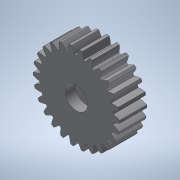
# Autodesk Inventor part: small-gear
Saved by Autodesk Inventor 2020 (Build 240168000, 168)
## iProperties
Created: 2020-05-22
Part Number: small-gear
Material: Ogólny
Document SubType Name: Modeling
Designer: blep
Density: 1 g/cm^3
Appearance: Domyślna
Author: blep
Autodesk Inventor part; units mm, degrees
ref_plane "YZ Plane" through (0, 0, 0) normal (1, 0, 0) x (0, 1, 0)
ref_plane "XZ Plane" through (0, 0, 0) normal (0, 1, 0) x (-1, 0, 0)
ref_plane "XY Plane" through (0, 0, 0) normal (0, 0, 1) x (1, 0, 0)
sketch "Szkic1" plane through (0, 0, 0) normal (0, 0, 1) x (1, 0, 0)
  arc A0 (-1.732, -4.0613) -> (-1.6613, -4.132) centre (0, -2.4) ccw projected
  arc A1 (0.05, -0.4006) -> (-0.05, -0.4006) centre (0, -2.4) ccw projected
  arc A2 (-0.05, -0.4006) -> (-0.5703, -0.483) centre (0, -2.4) ccw projected
  arc A3 (-0.5703, -0.483) -> (-0.6654, -0.5139) centre (0, -2.4) ccw projected
  arc A4 (-0.6654, -0.5139) -> (-1.1348, -0.7531) centre (0, -2.4) ccw projected
  arc A5 (-1.1348, -0.7531) -> (-1.2157, -0.8119) centre (0, -2.4) ccw projected
  arc A6 (-1.2157, -0.8119) -> (-1.5881, -1.1843) centre (0, -2.4) ccw projected
  arc A7 (-1.5881, -1.1843) -> (-1.6469, -1.2652) centre (0, -2.4) ccw projected
  arc A8 (-1.6469, -1.2652) -> (-1.8861, -1.7346) centre (0, -2.4) ccw projected
  arc A9 (-1.8861, -1.7346) -> (-1.917, -1.8297) centre (0, -2.4) ccw projected
  arc A10 (-1.917, -1.8297) -> (-1.9994, -2.35) centre (0, -2.4) ccw projected
  arc A11 (-1.9994, -2.35) -> (-1.9994, -2.45) centre (0, -2.4) ccw projected
  arc A12 (-1.9994, -2.45) -> (-1.917, -2.9703) centre (0, -2.4) ccw projected
  arc A13 (-1.917, -2.9703) -> (-1.8861, -3.0654) centre (0, -2.4) ccw projected
  arc A14 (-1.8861, -3.0654) -> (-1.6469, -3.5348) centre (0, -2.4) ccw projected
  arc A15 (-1.6469, -3.5348) -> (-1.5881, -3.6157) centre (0, -2.4) ccw projected
  arc A16 (-1.5881, -3.6157) -> (-1.2157, -3.9881) centre (0, -2.4) ccw projected
  arc A17 (-1.2157, -3.9881) -> (-1.1348, -4.0469) centre (0, -2.4) ccw projected
  arc A18 (-1.1348, -4.0469) -> (-0.6654, -4.2861) centre (0, -2.4) ccw projected
  arc A19 (-0.6654, -4.2861) -> (-0.5703, -4.317) centre (0, -2.4) ccw projected
  arc A20 (-0.5703, -4.317) -> (-0.05, -4.3994) centre (0, -2.4) ccw projected
  arc A21 (-0.05, -4.3994) -> (0.05, -4.3994) centre (0, -2.4) ccw projected
  arc A22 (0.05, -4.3994) -> (0.5703, -4.317) centre (0, -2.4) ccw projected
  arc A23 (0.5703, -4.317) -> (0.6654, -4.2861) centre (0, -2.4) ccw projected
  arc A24 (0.6654, -4.2861) -> (1.1348, -4.0469) centre (0, -2.4) ccw projected
  arc A25 (1.1348, -4.0469) -> (1.2157, -3.9881) centre (0, -2.4) ccw projected
  arc A26 (1.2157, -3.9881) -> (1.5881, -3.6157) centre (0, -2.4) ccw projected
  arc A27 (1.5881, -3.6157) -> (1.6469, -3.5348) centre (0, -2.4) ccw projected
  arc A28 (1.6469, -3.5348) -> (1.8861, -3.0654) centre (0, -2.4) ccw projected
  arc A29 (1.8861, -3.0654) -> (1.917, -2.9703) centre (0, -2.4) ccw projected
  arc A30 (1.917, -2.9703) -> (1.9994, -2.45) centre (0, -2.4) ccw projected
  arc A31 (1.9994, -2.45) -> (1.9994, -2.35) centre (0, -2.4) ccw projected
  arc A32 (1.9994, -2.35) -> (1.917, -1.8297) centre (0, -2.4) ccw projected
  arc A33 (1.917, -1.8297) -> (1.8861, -1.7346) centre (0, -2.4) ccw projected
  arc A34 (1.8861, -1.7346) -> (1.6469, -1.2652) centre (0, -2.4) ccw projected
  arc A35 (1.6469, -1.2652) -> (1.5881, -1.1843) centre (0, -2.4) ccw projected
  arc A36 (1.5881, -1.1843) -> (1.2157, -0.8119) centre (0, -2.4) ccw projected
  arc A37 (1.2157, -0.8119) -> (1.1348, -0.7531) centre (0, -2.4) ccw projected
  arc A38 (1.1348, -0.7531) -> (0.6654, -0.5139) centre (0, -2.4) ccw projected
  arc A39 (0.6654, -0.5139) -> (0.5703, -0.483) centre (0, -2.4) ccw projected
  arc A40 (0.5703, -0.483) -> (0.05, -0.4006) centre (0, -2.4) ccw projected
  circle A41 centre (0, -2.4) radius 1.5065 projected
  circle A42 centre (0, -2.4) radius 2.4
  circle A43 centre (0, -2.4) radius 15
  circle A44 centre (0, -2.4) radius 1.0065 projected
  circle A45 centre (0, -2.4) radius 1.2565
  circle A46 centre (0, -2.4) radius 2.9
  point P0 (0, 0)
  point P1 (-1.6613, -4.132)
  point P2 (-1.732, -4.0613)
  dimension "d0" = 30
  dimension "d3" = 0.25
  dimension "d12" = 0.5
  constraints: 4 centre point, 2 coincident, 1 concentric
  measures "d0" diameter of A43
  measures "d3" radial gap between concentric circles of A44 A45
  measures "d12" radial gap between concentric circles of A42 A46
extrude "Wyciągnięcie proste1" add sketch "Szkic1" against normal blind 3 contours A43
extrude "Wyciągnięcie proste2" add sketch "Szkic1" along normal blind 1.5 contours A42 A0 | A40 A39 A38 A37 A36 A35 A34 A33 A32 A31 A30 A29 A28 A27 A26 A25 A24 A23 A22 A21 A20 A19 A18 A17 A16 A15 A14 A13 A12 A11 A10 A9 A8 A7 A6 A5 A4 A3 A2 A1 | A41 | A43 | A45 | A46
sketch "Szkic2" plane through (0, -2.4, 1.5) normal (0, 0, 1) x (1, 0, 0)
  circle A0 centre (0, 0) radius 1.0065 projected
  circle A1 centre (0, 0) radius 3
  circle A2 centre (0, 0) radius 15 projected
  point P0 (0, 2.4)
  dimension "d6" = 6
  constraints: 1 centre point, 1 coincident
  measures "d6" diameter of A1
extrude "Wyciągnięcie proste3" add sketch "Szkic2" along normal blind 2.7 contours A2
sketch "Szkic4" plane through (0, -2.4, -3) normal (0, 0, -1) x (-1, 0, 0)
  arc A0 (4.4308, -8.6273) -> (5.208, -8.1816) centre (0, 0) ccw projected
  arc A1 (1.0151, -9.6453) -> (1.9007, -9.5105) centre (0, 0) ccw projected
  arc A2 (-2.5377, -9.3607) -> (-1.6632, -9.5549) centre (0, 0) ccw projected
  arc A3 (-5.7478, -7.8118) -> (-5.0025, -8.3088) centre (0, 0) ccw projected
  arc A4 (-8.1816, -5.208) -> (-7.6662, -5.9407) centre (0, 0) ccw projected
  arc A5 (-9.5105, -1.9007) -> (-9.2945, -2.7701) centre (0, 0) ccw projected
  arc A6 (-9.5549, 1.6632) -> (-9.6676, 0.7745) centre (0, 0) ccw projected
  arc A7 (-8.3088, 5.0025) -> (-8.735, 4.2145) centre (0, 0) ccw projected
  arc A8 (-5.9407, 7.6662) -> (-6.6227, 7.0854) centre (0, 0) ccw projected
  arc A9 (7.8118, -5.7478) -> (6.4204, -3.8655) centre (1.2511, -9.1422) ccw projected
  arc A10 (6.4204, -3.8655) -> (6.7497, -3.2567) centre (0, 0) ccw projected
  arc A11 (6.7497, -3.2567) -> (9.0866, -3.3906) centre (8.3355, 3.958) ccw projected
  arc A12 (9.0866, -3.3906) -> (9.3607, -2.5377) centre (0, 0) ccw projected
  arc A13 (9.3607, -2.5377) -> (7.3833, -1.2852) centre (4.4691, -8.0729) ccw projected
  arc A14 (7.3833, -1.2852) -> (7.4703, -0.5985) centre (0, 0) ccw projected
  arc A15 (7.4703, -0.5985) -> (9.6978, 0.1208) centre (6.3428, 6.7018) ccw projected
  arc A16 (9.6978, 0.1208) -> (9.6453, 1.0151) centre (0, 0) ccw projected
  arc A17 (9.6453, 1.0151) -> (7.3489, 1.4687) centre (7.0836, -5.9134) ccw projected
  arc A18 (7.3489, 1.4687) -> (7.1821, 2.1405) centre (0, 0) ccw projected
  arc A19 (7.1821, 2.1405) -> (8.9993, 3.6159) centre (3.4935, 8.5406) ccw projected
  arc A20 (8.9993, 3.6159) -> (8.6273, 4.4308) centre (0, 0) ccw projected
  arc A21 (8.6273, 4.4308) -> (6.3221, 4.0243) centre (8.7414, -2.9551) ccw projected
  arc A22 (6.3221, 4.0243) -> (5.9238, 4.5905) centre (0, 0) ccw projected
  arc A23 (5.9238, 4.5905) -> (7.0854, 6.6227) centre (0.1724, 9.2258) ccw projected
  arc A24 (7.0854, 6.6227) -> (6.4441, 7.2482) centre (0, 0) ccw projected
  arc A25 (6.4441, 7.2482) -> (4.4415, 6.0364) centre (9.2187, 0.4022) ccw projected
  arc A26 (4.4415, 6.0364) -> (3.8655, 6.4204) centre (0, 0) ccw projected
  arc A27 (3.8655, 6.4204) -> (4.2145, 8.735) centre (-3.172, 8.6651) ccw projected
  arc A28 (4.2145, 8.735) -> (3.3906, 9.0866) centre (0, 0) ccw projected
  arc A29 (3.3906, 9.0866) -> (1.9609, 7.2332) centre (8.4509, 3.7052) ccw projected
  arc A30 (1.9609, 7.2332) -> (1.2852, 7.3833) centre (0, 0) ccw projected
  arc A31 (1.2852, 7.3833) -> (0.7745, 9.6676) centre (-6.088, 6.9341) ccw projected
  arc A32 (0.7745, 9.6676) -> (-0.1208, 9.6978) centre (0, 0) ccw projected
  arc A33 (-0.1208, 9.6978) -> (-0.7844, 7.4531) centre (6.5417, 6.5078) ccw projected
  arc A34 (-0.7844, 7.4531) -> (-1.4687, 7.3489) centre (0, 0) ccw projected
  arc A35 (-1.4687, 7.3489) -> (-2.7701, 9.2945) centre (-8.1818, 4.2666) ccw projected
  arc A36 (-2.7701, 9.2945) -> (-3.6159, 8.9993) centre (0, 0) ccw projected
  arc A37 (-3.6159, 8.9993) -> (-3.4238, 6.6665) centre (3.7491, 8.4315) ccw projected
  arc A38 (-3.4238, 6.6665) -> (-4.0243, 6.3221) centre (0, 0) ccw projected
  arc A39 (-4.0243, 6.3221) -> (-5.9407, 7.6662) centre (-9.1706, 1.0229) ccw projected
  arc A40 (-6.6227, 7.0854) -> (-5.6008, 4.9795) centre (0.4501, 9.2165) ccw projected
  arc A41 (-5.6008, 4.9795) -> (-6.0364, 4.4415) centre (0, 0) ccw projected
  arc A42 (-6.0364, 4.4415) -> (-8.3088, 5.0025) centre (-8.9208, -2.359) ccw projected
  arc A43 (-8.735, 4.2145) -> (-7.0214, 2.62) centre (-2.9097, 8.7567) ccw projected
  arc A44 (-7.0214, 2.62) -> (-7.2332, 1.9609) centre (0, 0) ccw projected
  arc A45 (-7.2332, 1.9609) -> (-9.5549, 1.6632) centre (-7.4663, -5.4222) ccw projected
  arc A46 (-9.6676, 0.7745) -> (-7.4937, -0.0934) centre (-5.8765, 7.1143) ccw projected
  arc A47 (-7.4937, -0.0934) -> (-7.4531, -0.7844) centre (0, 0) ccw projected
  arc A48 (-7.4531, -0.7844) -> (-9.5105, -1.9007) centre (-5.0034, -7.7532) ccw projected
  arc A49 (-9.2945, -2.7701) -> (-6.9539, -2.7941) centre (-8.0496, 4.5111) ccw projected
  arc A50 (-6.9539, -2.7941) -> (-6.6665, -3.4238) centre (0, 0) ccw projected
  arc A51 (-6.6665, -3.4238) -> (-8.1816, -5.208) centre (-1.8647, -9.0371) ccw projected
  arc A52 (-7.6662, -5.9407) -> (-5.475, -5.1175) centre (-9.1356, 1.2986) ccw projected
  arc A53 (-5.475, -5.1175) -> (-4.9795, -5.6008) centre (0, 0) ccw projected
  arc A54 (-4.9795, -5.6008) -> (-5.7478, -7.8118) centre (1.5258, -9.1004) ccw projected
  arc A55 (-5.0025, -8.3088) -> (-3.2567, -6.7497) centre (-8.9878, -2.0893) ccw projected
  arc A56 (-3.2567, -6.7497) -> (-2.62, -7.0214) centre (0, 0) ccw projected
  arc A57 (-2.62, -7.0214) -> (-2.5377, -9.3607) centre (4.7102, -7.9347) ccw projected
  arc A58 (-1.6632, -9.5549) -> (-0.5985, -7.4703) centre (-7.6261, -5.195) ccw projected
  arc A59 (-0.5985, -7.4703) -> (0.0934, -7.4937) centre (0, 0) ccw projected
  arc A60 (0.0934, -7.4937) -> (1.0151, -9.6453) centre (7.2585, -5.6974) ccw projected
  arc A61 (1.9007, -9.5105) -> (2.1405, -7.1821) centre (-5.2345, -7.599) ccw projected
  arc A62 (2.1405, -7.1821) -> (2.7941, -6.9539) centre (0, 0) ccw projected
  arc A63 (2.7941, -6.9539) -> (4.4308, -8.6273) centre (8.8265, -2.6906) ccw projected
  arc A64 (5.208, -8.1816) -> (4.5905, -5.9238) centre (-2.136, -8.9768) ccw projected
  arc A65 (4.5905, -5.9238) -> (5.1175, -5.475) centre (0, 0) ccw projected
  arc A66 (5.1175, -5.475) -> (7.2482, -6.4441) centre (9.2024, 0.6796) ccw projected
  arc A67 (7.2482, -6.4441) -> (7.8118, -5.7478) centre (0, 0) ccw projected
  point P0 (0, 2.4)
  point P1 (0, 0)
extrude "Wyciągnięcie proste5" cut sketch "Szkic4" against normal blind 10 keep common part
